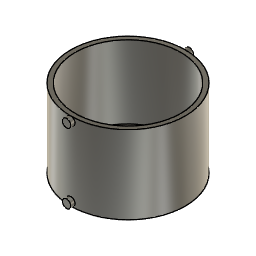
PipeCapCoupler (Autodesk Fusion 360 design; units mm, degrees)
Autodesk Fusion 360 part; units mm, degrees
note: some values were not read from the file. Chosen so that the rebuilt part matches the saved one: which face or edge a step refers to; where a step ends.
sketch "Sketch1" plane through (0, 0, 0) normal (0, 0, 1) x (1, 0, 0)
  circle A0 centre (0, 0) radius 22
  dimension "d1" = 44
  constraint coincident A0.centre origin
  measures "d1" diameter of A0
extrude "Extrude1" add sketch "Sketch1" along normal blind 30
sketch "Sketch2" plane through (0, 0, 30) normal (0, 0, 1) x (-1, 0, 0)
  circle A0 centre (0, 0) radius 22
  circle A1 centre (0, 0) radius 20.3
  dimension "d4" = 40.6
  constraint coincident A0.centre A1.centre
  measures "d4" diameter of A1
extrude "Extrude2" cut sketch "Sketch2" against normal blind 28 contours A1
ref_plane "WorkPlane2" through (0, 22, 0) normal (0, 1, 0) x (0, 0, 1)
sketch "Sketch8" plane through (0, 22, 0) normal (0, 1, 0) x (1, 0, 0)
  circle A0 centre (0, -1.6) radius 1.6
  line L0 (-22, 0) -> (22, 0)
  dimension "d29" = 3.2
  dimension "d32" = 1.6
  measures "d29" diameter of A0
  measures "d32" distance of A0.centre L0
extrude "Extrude7" add sketch "Sketch8" along normal blind 1.6 and the other way up to near side of body 1
mirror "Mirror1" about plane through (0, 0, 0) normal (0, 1, 0) of bodies 1 merged
ref_plane "WorkPlane3" through (0, 0, 15) normal (0, 0, -1) x (-1, 0, 0)
mirror "Mirror2" about plane through (0, 0, 15) normal (0, 0, -1) of 4 faces at (-1.5948, 23.0474, 1.7285) (-1.5948, -23.0474, 1.7285) (0.0844, 23.6, 2.231) (0.0844, -23.6, 2.231)
equation "d1 = LowerOuterDiam"
equation "d4 = LowerInnerDiam + PipeTol"
equation "PipeTol = 0.6 mm"
equation "LowerInnerDiam = 40 mm"
equation "LowerOuterDiam = 44 mm"
equation "d28 = LowerOuterDiam / 2"
equation "d29 = AnchorDiam"
equation "AnchorDiam = 3.2 mm"
equation "AnchorFillet = 3 mm"
equation "d32 = AnchorDiam / 2"
equation "d33 = AnchorDiam / 2"
